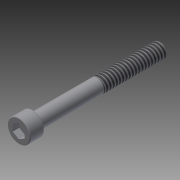
# Autodesk Inventor part: D-D0144-SS-1-bif
Saved by Autodesk Inventor 2014 SP2 (Build 180246200, 246)
## iProperties
Created: 2020-02-04
Part Number: D-D0144-SS-1-bif
Material: Generic
Catalog Web Link: www.cadenas.de
Description: BIF Screw-Bimba FLAT-1
Vendor: BIMBA
Document SubType Name: Modeling
Designer: psadmin
Manufacturer: BIMBA
Mass: 0.199603 g
Surface Area: 3.05763 cm^2
Volume: 0.199603 cm^3
Density: 1 g/cm^3
Appearance: PSOLRGB-192-192-192
Category: PARTsolutions
Company: BIMBA
Title: D-D0144-SS-1-bif
Author: Cadenas PARTsolutions
Comments: Bimba FLAT-1
PSOL_IDENT_0: {$CADENAS_DATA\23d-libs\bimba\bimba_brand\bimba_imperial\bimba_full_line\flat_cylinders\fo1\bif_scre
PSOL_IDENT_1: w.prj},177 {VTYP=3D},{NB=D-D0144-SS-1-bif},{LINA=D-D0144-SS-1-bif},{NN=BIF Screw},{DATE=22.01.2020 0
PSOL_IDENT_2: 9:06:04},{GEOMDATE=09.03.2017 10:16:43},{VERSION=},{LINEID=10},{WBVAR=L},{WBNUMERIC=L}  {NB=D-D0144-
PSOL_IDENT_3: SS-1-bif},{LINA=D-D0144-SS-1-bif},{KT=DUMMY},{PN=D-D0144-SS-1},{MODEL=D-D0144-SS},{NDM=0.112},{L=1.0
PSOL_IDENT_4: 0000},{H=0.179},{HL=0.110},{HW=0.09400},{HWL=0.051},{CH=0.005}
NN: BIF Screw
NT: Bimba FLAT-1
NB: D-D0144-SS-1-bif
NBSYN: $PN.-bif
LINA: D-D0144-SS-1-bif
PN: D-D0144-SS-1
MODEL: D-D0144-SS
NDM: 0.112
L: 1
H: 0.179
HL: 0.11
HW: 0.094
HWL: 0.051
CH: 0.005
SUPPLIER: BIMBA
ARTICLENO: D-D0144-SS-1-bif
BOMINFO: D-D0144-SS-1-bif
CREATOR: CADENAS GmbH
Autodesk Inventor part; units mm, degrees
sketch "Sketch_1" plane through (0, 0, 0) normal (1, 0, 0) x (0, 1, 0)
  line L0 (0, -28.194) -> (0, 0)
  line L1 (0, 0) -> (2.1463, 0)
  line L2 (2.1463, 0) -> (2.2733, -0.127)
  line L3 (2.2733, -0.127) -> (2.2733, -2.667)
  line L4 (2.2733, -2.667) -> (2.1463, -2.794)
  line L5 (2.1463, -2.794) -> (1.4224, -2.794)
  line L6 (1.4224, -2.794) -> (1.4224, -27.8155)
  line L7 (1.4224, -27.8155) -> (1.0439, -28.194)
  line L8 (1.0439, -28.194) -> (0, -28.194)
  line L9 (0, -28.194) -> (0, 0)
  constraints: 20 end point
revolve "Revolution1" add sketch "Sketch_1" angle 360 about axis through (0, 0, -28.194) along (0, 0, -1)
thread "Thread1" size "4-40 UNC" class "2A" standard "ANSI Unified Screw Threads" length 12.3215
sketch "Sketch_3" plane through (0, 0, 0) normal (0, 0, 1) x (1, 0, 0)
  line L0 (-1.1938, -0.6892) -> (0, -1.3785)
  line L1 (0, -1.3785) -> (1.1938, -0.6892)
  line L2 (1.1938, -0.6892) -> (1.1938, 0.6892)
  line L3 (1.1938, 0.6892) -> (0, 1.3785)
  line L4 (0, 1.3785) -> (-1.1938, 0.6892)
  line L5 (-1.1938, 0.6892) -> (-1.1938, -0.6892)
  constraints: 12 end point
extrude "Extrusion1" cut sketch "Sketch_3" against normal blind 1.2954
ref_plane "screw_XY" through (0, 0, -2.794) normal (0, 0, 1) x (1, 0, 0)
ref_plane "screw_YZ" through (0, 0, -2.794) normal (1, 0, 0) x (0, 1, 0)
ref_plane "screw_ZX" through (0, 0, -2.794) normal (0, 1, 0) x (0, 0, 1)
body "Solid1"
